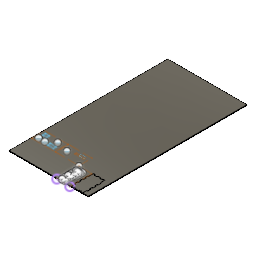
generated POWER BOX  6 CUT first v1 (Autodesk Fusion 360 design; units mm, degrees)
Autodesk Fusion 360 part; units mm, degrees
sketch "b top content" plane through (0, 0, 0) normal (0, 0, 1) x (1, 0, 0)
  line L0 (0, 85) -> (90, 85) construction
  line L1 (90, 0) -> (0, 0) construction
  line L2 (14.1663, 44.1604) -> (78.1663, 44.1604) construction
  line L3 (78.1663, 44.1604) -> (78.1663, 63.1604) construction
  line L4 (78.1663, 63.1604) -> (14.1663, 63.1604) construction
  line L5 (14.1663, 63.1604) -> (14.1663, 44.1604) construction
  line L6 (0, 0) -> (0, 85) construction
  dimension "d1818" = 15
  dimension "d1163" = 90
  dimension "d1817" = 85
  constraint horizontal L0
  constraint perpendicular L1 L6
  measures "d1163" distance of L0.start L0.end
  measures "d1817" distance of L1.start L0.end
sketch "b front content" plane through (0, 0, 0) normal (0, 0, 1) x (1, 0, 0)
  line L0 (53.5, 95.01) -> (53.5, 105.31)
  circle A0 centre (13, 101.01) radius 6
  circle A1 centre (37, 101.01) radius 6
  line L1 (76.2, 105.31) -> (76.2, 95.01)
  line L2 (26.5, 128.31) -> (26.5, 118.01)
  line L3 (26.5, 118.01) -> (12, 118.01)
  line L4 (90, 137.01) -> (0, 137.01) construction
  circle A2 centre (65, 122.51) radius 3.5
  line L5 (76.2, 95.01) -> (53.5, 95.01)
  line L6 (53.5, 105.31) -> (76.2, 105.31)
  line L7 (90, 87.01) -> (90, 137.01) construction
  line L8 (0, 87.01) -> (0, 137.01) construction
  line L9 (12, 128.31) -> (26.5, 128.31)
  line L10 (12, 118.01) -> (12, 128.31)
  line L11 (0, 87.01) -> (90, 87.01) construction
  dimension "d230" = 90
  dimension "d231" = 50
  dimension "d232" = 12
  dimension "d233" = 24
  dimension "d234" = 14
  dimension "d235" = 13
  dimension "d236" = 14.5
  dimension "d237" = 10.3
  dimension "d238" = 31
  dimension "d239" = 12
  dimension "d240" = 7
  dimension "d241" = 25
  dimension "d242" = 14.5
  dimension "d243" = 22.7
  dimension "d244" = 10.3
  dimension "d245" = 13.8
  dimension "d246" = 8
  constraint perpendicular L4 L8
  constraint equal A0 A1
  measures "d230" distance of L7.start L8.start
  measures "d231" distance of L8.start L4.end
  measures "d232" diameter of A1
  measures "d233" distance of A1.centre A0.centre
  measures "d234" distance of A1.centre L11
  measures "d235" distance of A0.centre L8
  measures "d236" distance of L2.end L3.end
  measures "d237" distance of L2.end L2.start
  measures "d238" distance of L3 L11
  measures "d239" distance of L8 L10
  measures "d240" diameter of A2
  measures "d241" distance of A2.centre L7
  measures "d242" distance of A2.centre L4
  measures "d243" distance of L1.end L0.start
  measures "d244" distance of L1.start L1.end
  measures "d245" distance of L1 L7
  measures "d246" distance of L5 L11
sketch " b back content" plane through (0, 0, 0) normal (0, 0, 1) x (1, 0, 0)
  line L0 (182.01, 87.01) -> (182.01, 137.01) construction
  line L1 (182.01, 137.01) -> (92.01, 137.01) construction
  circle A0 centre (110.81, 112.01) radius 4
  line L2 (92.01, 137.01) -> (92.01, 87.01) construction
  line L3 (169.3373, 123.3571) -> (135.0459, 123.3571) construction
  line L4 (135.0459, 123.3571) -> (135.0459, 117.5676) construction
  line L5 (135.0459, 117.5676) -> (169.3373, 117.5676) construction
  line L6 (169.3373, 117.5676) -> (169.3373, 123.3571) construction
  line L7 (92.01, 87.01) -> (182.01, 87.01) construction
  point P0 (184.02, 85)
  dimension "d1816" = 5
  dimension "d502" = 90
  dimension "d503" = 50
  dimension "d696" = 25
  dimension "d1179" = 18.8
  dimension "d1562" = 8
  measures "d502" distance of L1.end L0.end
  measures "d503" distance of L0.start L0.end
  measures "d696" distance of A0.centre L1
  measures "d1179" distance of A0.centre L2
  measures "d1562" diameter of A0
sketch "b  stock" plane through (0, 0, 0) normal (0, 0, 1) x (1, 0, 0)
  line L0 (0, 0) -> (304.8, 0)
  line L1 (304.8, 0) -> (304.8, 609.6)
  line L2 (304.8, 609.6) -> (0, 609.6)
  line L3 (0, 609.6) -> (0, 0)
extrude "b  stock body extrude Feature" add sketch "b  stock" along normal blind 3.175 makes body 1
sketch "b  layout" plane through (0, 0, 0) normal (0, 0, 1) x (1, 0, 0)
  line L0 (0, 0) -> (90, 0)
  line L1 (90, 0) -> (90, 85)
  line L2 (90, 85) -> (0, 85)
  line L3 (0, 85) -> (0, 0)
  line L4 (92.01, 0) -> (182.01, 0)
  line L5 (182.01, 0) -> (182.01, 85)
  line L6 (182.01, 85) -> (92.01, 85)
  line L7 (92.01, 85) -> (92.01, 0)
  line L8 (184.02, 0) -> (234.02, 0)
  line L9 (234.02, 0) -> (234.02, 85)
  line L10 (234.02, 85) -> (184.02, 85)
  line L11 (184.02, 85) -> (184.02, 0)
  line L12 (236.03, 0) -> (286.03, 0)
  line L13 (286.03, 0) -> (286.03, 85)
  line L14 (286.03, 85) -> (236.03, 85)
  line L15 (236.03, 85) -> (236.03, 0)
  line L16 (0, 87.01) -> (90, 87.01)
  line L17 (90, 87.01) -> (90, 137.01)
  line L18 (90, 137.01) -> (0, 137.01)
  line L19 (0, 137.01) -> (0, 87.01)
  line L20 (92.01, 87.01) -> (182.01, 87.01)
  line L21 (182.01, 87.01) -> (182.01, 137.01)
  line L22 (182.01, 137.01) -> (92.01, 137.01)
  line L23 (92.01, 137.01) -> (92.01, 87.01)
sketch "b top lines" plane through (0, 0, 0) normal (0, 0, 1) x (1, 0, 0)
  line L0 (0, 0) -> (10.15, 0)
  line L1 (10.15, 0) -> (10.15, 3.175)
  line L2 (10.15, 3.175) -> (19.85, 3.175)
  line L3 (19.85, 3.175) -> (19.85, 0)
  line L4 (19.85, 0) -> (30.15, 0)
  line L5 (30.15, 0) -> (30.15, 3.175)
  line L6 (30.15, 3.175) -> (39.85, 3.175)
  line L7 (39.85, 3.175) -> (39.85, 0)
  line L8 (39.85, 0) -> (50.15, 0)
  line L9 (50.15, 0) -> (50.15, 3.175)
  line L10 (50.15, 3.175) -> (59.85, 3.175)
  line L11 (59.85, 3.175) -> (59.85, 0)
  line L12 (59.85, 0) -> (70.15, 0)
  line L13 (70.15, 0) -> (70.15, 3.175)
  line L14 (70.15, 3.175) -> (79.85, 3.175)
  line L15 (79.85, 3.175) -> (79.85, 0)
  line L16 (79.85, 0) -> (90, 0)
  line L17 (90, 0) -> (90, 17.65)
  line L18 (90, 17.65) -> (86.825, 17.65)
  line L19 (86.825, 17.65) -> (86.825, 27.35)
  line L20 (86.825, 27.35) -> (90, 27.35)
  line L21 (90, 27.35) -> (90, 37.65)
  line L22 (90, 37.65) -> (86.825, 37.65)
  line L23 (86.825, 37.65) -> (86.825, 47.35)
  line L24 (86.825, 47.35) -> (90, 47.35)
  line L25 (90, 47.35) -> (90, 57.65)
  line L26 (90, 57.65) -> (86.825, 57.65)
  line L27 (86.825, 57.65) -> (86.825, 67.35)
  line L28 (86.825, 67.35) -> (90, 67.35)
  line L29 (90, 67.35) -> (90, 85)
  line L30 (0, 85) -> (10.15, 85)
  line L31 (10.15, 85) -> (10.15, 81.825)
  line L32 (10.15, 81.825) -> (19.85, 81.825)
  line L33 (19.85, 81.825) -> (19.85, 85)
  line L34 (19.85, 85) -> (30.15, 85)
  line L35 (30.15, 85) -> (30.15, 81.825)
  line L36 (30.15, 81.825) -> (39.85, 81.825)
  line L37 (39.85, 81.825) -> (39.85, 85)
  line L38 (39.85, 85) -> (50.15, 85)
  line L39 (50.15, 85) -> (50.15, 81.825)
  line L40 (50.15, 81.825) -> (59.85, 81.825)
  line L41 (59.85, 81.825) -> (59.85, 85)
  line L42 (59.85, 85) -> (70.15, 85)
  line L43 (70.15, 85) -> (70.15, 81.825)
  line L44 (70.15, 81.825) -> (79.85, 81.825)
  line L45 (79.85, 81.825) -> (79.85, 85)
  line L46 (79.85, 85) -> (90, 85)
  line L47 (0, 0) -> (0, 17.65)
  line L48 (0, 17.65) -> (3.175, 17.65)
  line L49 (3.175, 17.65) -> (3.175, 27.35)
  line L50 (3.175, 27.35) -> (0, 27.35)
  line L51 (0, 27.35) -> (0, 37.65)
  line L52 (0, 37.65) -> (3.175, 37.65)
  line L53 (3.175, 37.65) -> (3.175, 47.35)
  line L54 (3.175, 47.35) -> (0, 47.35)
  line L55 (0, 47.35) -> (0, 57.65)
  line L56 (0, 57.65) -> (3.175, 57.65)
  line L57 (3.175, 57.65) -> (3.175, 67.35)
  line L58 (3.175, 67.35) -> (0, 67.35)
  line L59 (0, 67.35) -> (0, 85)
sketch "b top circles" plane through (0, 0, 0) normal (0, 0, 1) x (1, 0, 0)
  circle A0 centre (10.6806, 2.4644) radius 1.005
  circle A1 centre (19.3194, 2.4644) radius 1.005
  circle A2 centre (30.6806, 2.4644) radius 1.005
  circle A3 centre (39.3194, 2.4644) radius 1.005
  circle A4 centre (50.6806, 2.4644) radius 1.005
  circle A5 centre (59.3194, 2.4644) radius 1.005
  circle A6 centre (70.6806, 2.4644) radius 1.005
  circle A7 centre (79.3194, 2.4644) radius 1.005
  circle A8 centre (87.5356, 18.1806) radius 1.005
  circle A9 centre (87.5356, 26.8194) radius 1.005
  circle A10 centre (87.5356, 38.1806) radius 1.005
  circle A11 centre (87.5356, 46.8194) radius 1.005
  circle A12 centre (87.5356, 58.1806) radius 1.005
  circle A13 centre (87.5356, 66.8194) radius 1.005
  circle A14 centre (10.6806, 82.5356) radius 1.005
  circle A15 centre (19.3194, 82.5356) radius 1.005
  circle A16 centre (30.6806, 82.5356) radius 1.005
  circle A17 centre (39.3194, 82.5356) radius 1.005
  circle A18 centre (50.6806, 82.5356) radius 1.005
  circle A19 centre (59.3194, 82.5356) radius 1.005
  circle A20 centre (70.6806, 82.5356) radius 1.005
  circle A21 centre (79.3194, 82.5356) radius 1.005
  circle A22 centre (2.4644, 18.1806) radius 1.005
  circle A23 centre (2.4644, 26.8194) radius 1.005
  circle A24 centre (2.4644, 38.1806) radius 1.005
  circle A25 centre (2.4644, 46.8194) radius 1.005
  circle A26 centre (2.4644, 58.1806) radius 1.005
  circle A27 centre (2.4644, 66.8194) radius 1.005
extrude "b top lines lines extrude Feature" add sketch "b top lines" along normal blind 3.175 separate body makes body 2
extrude "b top circles circles extrude Feature" add sketch "b top circles" along normal blind 3.175 separate body makes body 3 at (3.4644, 58.0806, 2.1167) makes body 4 at (3.4644, 38.0806, 2.1167) makes body 5 at (3.4644, 18.0806, 2.1167) makes body 6 at (69.7363, 82.8794, 2.1167) makes body 7 at (49.7363, 82.8794, 2.1167) makes body 8 at (31.6067, 82.926, 2.1167) makes body 9 at (9.7363, 82.8794, 2.1167) makes body 10 at (86.5913, 67.1631, 2.1167) makes body 11 at (87.2156, 45.8667, 1.0583) makes body 12 at (87.2156, 25.8667, 1.0583) makes body 13 at (78.9993, 1.5117, 1.0583) makes body 14 at (59.2943, 3.469, 2.1167) makes body 15 at (39.2943, 3.469, 2.1167) makes body 16 at (20.3194, 2.3643, 2.1167) makes body 17 at (31.6806, 2.3643, 2.1167) makes body 18 at (50.6556, 3.469, 2.1167) makes body 19 at (70.3606, 1.5117, 1.0583) makes body 20 at (87.2156, 17.228, 1.0583) makes body 21 at (87.2156, 37.228, 1.0583) makes body 22 at (87.2156, 57.228, 1.0583) makes body 23 at (11.6806, 2.3643, 2.1167) makes body 24 at (20.2454, 82.926, 2.1167) makes body 25 at (38.375, 82.8794, 2.1167) makes body 26 at (58.375, 82.8794, 2.1167) makes body 27 at (78.375, 82.8794, 2.1167) makes body 28 at (3.4644, 26.7193, 2.1167) makes body 29 at (3.4644, 46.7193, 2.1167) makes body 30 at (3.3904, 67.2097, 2.1167)
combine "b top lines final combine feature" operation cut target body 2 tool bodies 3 4 5 6 7 8 9 10 11 12 13 14 15 16 17 18 19 20 21 22 23 24 25 26 27 28 29 30
sketch "b bottom lines" plane through (0, 0, 0) normal (0, 0, 1) x (1, 0, 0)
  line L0 (92.01, 0) -> (102.16, 0)
  line L1 (102.16, 0) -> (102.16, 3.175)
  line L2 (102.16, 3.175) -> (111.86, 3.175)
  line L3 (111.86, 3.175) -> (111.86, 0)
  line L4 (111.86, 0) -> (122.16, 0)
  line L5 (122.16, 0) -> (122.16, 3.175)
  line L6 (122.16, 3.175) -> (131.86, 3.175)
  line L7 (131.86, 3.175) -> (131.86, 0)
  line L8 (131.86, 0) -> (142.16, 0)
  line L9 (142.16, 0) -> (142.16, 3.175)
  line L10 (142.16, 3.175) -> (151.86, 3.175)
  line L11 (151.86, 3.175) -> (151.86, 0)
  line L12 (151.86, 0) -> (162.16, 0)
  line L13 (162.16, 0) -> (162.16, 3.175)
  line L14 (162.16, 3.175) -> (171.86, 3.175)
  line L15 (171.86, 3.175) -> (171.86, 0)
  line L16 (171.86, 0) -> (182.01, 0)
  line L17 (182.01, 0) -> (182.01, 17.65)
  line L18 (182.01, 17.65) -> (178.835, 17.65)
  line L19 (178.835, 17.65) -> (178.835, 27.35)
  line L20 (178.835, 27.35) -> (182.01, 27.35)
  line L21 (182.01, 27.35) -> (182.01, 37.65)
  line L22 (182.01, 37.65) -> (178.835, 37.65)
  line L23 (178.835, 37.65) -> (178.835, 47.35)
  line L24 (178.835, 47.35) -> (182.01, 47.35)
  line L25 (182.01, 47.35) -> (182.01, 57.65)
  line L26 (182.01, 57.65) -> (178.835, 57.65)
  line L27 (178.835, 57.65) -> (178.835, 67.35)
  line L28 (178.835, 67.35) -> (182.01, 67.35)
  line L29 (182.01, 67.35) -> (182.01, 85)
  line L30 (92.01, 85) -> (102.16, 85)
  line L31 (102.16, 85) -> (102.16, 81.825)
  line L32 (102.16, 81.825) -> (111.86, 81.825)
  line L33 (111.86, 81.825) -> (111.86, 85)
  line L34 (111.86, 85) -> (122.16, 85)
  line L35 (122.16, 85) -> (122.16, 81.825)
  line L36 (122.16, 81.825) -> (131.86, 81.825)
  line L37 (131.86, 81.825) -> (131.86, 85)
  line L38 (131.86, 85) -> (142.16, 85)
  line L39 (142.16, 85) -> (142.16, 81.825)
  line L40 (142.16, 81.825) -> (151.86, 81.825)
  line L41 (151.86, 81.825) -> (151.86, 85)
  line L42 (151.86, 85) -> (162.16, 85)
  line L43 (162.16, 85) -> (162.16, 81.825)
  line L44 (162.16, 81.825) -> (171.86, 81.825)
  line L45 (171.86, 81.825) -> (171.86, 85)
  line L46 (171.86, 85) -> (182.01, 85)
  line L47 (92.01, 0) -> (92.01, 17.65)
  line L48 (92.01, 17.65) -> (95.185, 17.65)
  line L49 (95.185, 17.65) -> (95.185, 27.35)
  line L50 (95.185, 27.35) -> (92.01, 27.35)
  line L51 (92.01, 27.35) -> (92.01, 37.65)
  line L52 (92.01, 37.65) -> (95.185, 37.65)
  line L53 (95.185, 37.65) -> (95.185, 47.35)
  line L54 (95.185, 47.35) -> (92.01, 47.35)
  line L55 (92.01, 47.35) -> (92.01, 57.65)
  line L56 (92.01, 57.65) -> (95.185, 57.65)
  line L57 (95.185, 57.65) -> (95.185, 67.35)
  line L58 (95.185, 67.35) -> (92.01, 67.35)
  line L59 (92.01, 67.35) -> (92.01, 85)
sketch "b bottom circles" plane through (0, 0, 0) normal (0, 0, 1) x (1, 0, 0)
  circle A0 centre (102.6906, 2.4644) radius 1.005
  circle A1 centre (111.3294, 2.4644) radius 1.005
  circle A2 centre (122.6906, 2.4644) radius 1.005
  circle A3 centre (131.3294, 2.4644) radius 1.005
  circle A4 centre (142.6906, 2.4644) radius 1.005
  circle A5 centre (151.3294, 2.4644) radius 1.005
  circle A6 centre (162.6906, 2.4644) radius 1.005
  circle A7 centre (171.3294, 2.4644) radius 1.005
  circle A8 centre (179.5456, 18.1806) radius 1.005
  circle A9 centre (179.5456, 26.8194) radius 1.005
  circle A10 centre (179.5456, 38.1806) radius 1.005
  circle A11 centre (179.5456, 46.8194) radius 1.005
  circle A12 centre (179.5456, 58.1806) radius 1.005
  circle A13 centre (179.5456, 66.8194) radius 1.005
  circle A14 centre (102.6906, 82.5356) radius 1.005
  circle A15 centre (111.3294, 82.5356) radius 1.005
  circle A16 centre (122.6906, 82.5356) radius 1.005
  circle A17 centre (131.3294, 82.5356) radius 1.005
  circle A18 centre (142.6906, 82.5356) radius 1.005
  circle A19 centre (151.3294, 82.5356) radius 1.005
  circle A20 centre (162.6906, 82.5356) radius 1.005
  circle A21 centre (171.3294, 82.5356) radius 1.005
  circle A22 centre (94.4744, 18.1806) radius 1.005
  circle A23 centre (94.4744, 26.8194) radius 1.005
  circle A24 centre (94.4744, 38.1806) radius 1.005
  circle A25 centre (94.4744, 46.8194) radius 1.005
  circle A26 centre (94.4744, 58.1806) radius 1.005
  circle A27 centre (94.4744, 66.8194) radius 1.005
sketch "b bottom content" plane through (0, 0, 0) normal (0, 0, 1) x (1, 0, 0)
  line L0 (92.01, 0) -> (182.01, 0) construction
  line L1 (182.01, 0) -> (182.01, 85) construction
  line L2 (182.01, 85) -> (92.01, 85) construction
  line L3 (92.01, 85) -> (92.01, 0) construction
  line L4 (182.01, 85) -> (182.01, 0) construction
  line L5 (182.01, 0) -> (92.01, 0) construction
  line L6 (92.01, 85) -> (182.01, 85) construction
  line L7 (92.01, 0) -> (92.01, 85) construction
  circle A0 centre (108.01, 55.5) radius 1.005
  circle A1 centre (172.01, 75) radius 1.005
  circle A2 centre (166.01, 55.5) radius 1.005
  circle A3 centre (166.01, 29.5) radius 1.005
  circle A4 centre (172.01, 10) radius 1.005
  circle A5 centre (102.01, 10) radius 1.005
  circle A6 centre (108.01, 29.5) radius 1.005
  circle A7 centre (102.01, 75) radius 1.005
  circle A8 centre (172.01, 75) radius 1.005
  point P0 (102.01, 75)
  point P1 (108.01, 55.5)
  point P2 (172.01, 75)
  point P3 (166.01, 29.5)
  point P4 (166.01, 55.5)
  point P5 (172.01, 10)
  point P6 (102.01, 10)
  point P7 (108.01, 29.5)
  point P8 (182.01, 85)
  dimension "d467" = 90
  dimension "d468" = 85
  dimension "d469" = 10
  dimension "d470" = 10
  dimension "d471" = 29.5
  dimension "d472" = 16
  dimension "d473" = 2.01
  dimension "d474" = 2.01
  constraint horizontal L5
  constraint perpendicular L5 L7
  constraint parallel L5 L6
  constraint coincident L1.end L2.start
  constraint vertical L4
  constraint coincident P1 A0.centre
  constraint coincident P2 A1.centre
  constraint coincident P4 A2.centre
  constraint coincident P3 A3.centre
  constraint coincident P5 A4.centre
  constraint coincident P6 A5.centre
  constraint coincident P7 A6.centre
  constraint coincident P0 A7.centre
  constraint concentric A1 A8
  constraint equal A0 A2
  constraint equal A7 A8
  constraint equal A0 A6
  constraint equal A0 A3
  constraint equal A3 A5
  constraint equal A3 A8
  constraint equal A2 A4
  measures "d467" distance of L1.end L2.end
  measures "d468" distance of L0.start L2.end
  measures "d469" distance of P0 L6
  measures "d470" distance of P0 L7
  measures "d471" distance of P1 L6
  measures "d472" distance of P7 L7
  measures "d473" diameter of A0
  measures "d474" diameter of A1
extrude "b bottom lines lines extrude Feature" add sketch "b bottom lines" along normal blind 3.175 separate body makes body 31
extrude "b bottom circles circles extrude Feature" add sketch "b bottom circles" along normal blind 3.175 separate body makes body 32 at (94.1543, 57.228, 1.0583) makes body 33 at (94.1543, 37.228, 1.0583) makes body 34 at (94.1543, 17.228, 1.0583) makes body 35 at (161.7463, 82.8794, 2.1167) makes body 36 at (141.7463, 82.8794, 2.1167) makes body 37 at (121.7463, 82.8794, 2.1167) makes body 38 at (101.7463, 82.8794, 2.1167) makes body 39 at (178.6013, 67.1631, 2.1167) makes body 40 at (180.4717, 47.2097, 2.1167) makes body 41 at (179.959, 27.7354, 2.1167) makes body 42 at (170.916, 3.3804, 2.1167) makes body 43 at (150.916, 3.3804, 2.1167) makes body 44 at (130.916, 3.3804, 2.1167) makes body 45 at (111.0093, 1.5117, 1.0583) makes body 46 at (122.3706, 1.5117, 1.0583) makes body 47 at (142.2773, 3.3804, 2.1167) makes body 48 at (162.2773, 3.3804, 2.1167) makes body 49 at (179.959, 19.0967, 2.1167) makes body 50 at (180.4717, 38.571, 2.1167) makes body 51 at (180.4717, 58.571, 2.1167) makes body 52 at (102.3706, 1.5117, 1.0583) makes body 53 at (110.385, 82.8794, 2.1167) makes body 54 at (130.385, 82.8794, 2.1167) makes body 55 at (150.385, 82.8794, 2.1167) makes body 56 at (170.385, 82.8794, 2.1167) makes body 57 at (94.1543, 25.8667, 1.0583) makes body 58 at (94.1543, 45.8667, 1.0583) makes body 59 at (93.53, 67.1631, 2.1167)
combine "b bottom lines final combine feature" operation cut target body 31 tool bodies 32 33 34 35 36 37 38 39 40 41 42 43 44 45 46 47 48 49 50 51 52 53 54 55 56 57 58 59
sketch "b left lines" plane through (0, 0, 0) normal (0, 0, 1) x (1, 0, 0)
  line L0 (187.195, 0) -> (194.17, 0)
  line L1 (194.17, 0) -> (194.17, 3.175)
  line L2 (194.17, 3.175) -> (203.87, 3.175)
  line L3 (203.87, 3.175) -> (203.87, 0)
  line L4 (203.87, 0) -> (214.17, 0)
  line L5 (214.17, 0) -> (214.17, 3.175)
  line L6 (214.17, 3.175) -> (223.87, 3.175)
  line L7 (223.87, 3.175) -> (223.87, 0)
  line L8 (223.87, 0) -> (230.845, 0)
  line L9 (230.845, 0) -> (230.845, 17.35)
  line L10 (230.845, 17.35) -> (234.02, 17.35)
  line L11 (234.02, 17.35) -> (234.02, 27.65)
  line L12 (234.02, 27.65) -> (230.845, 27.65)
  line L13 (230.845, 27.65) -> (230.845, 37.35)
  line L14 (230.845, 37.35) -> (234.02, 37.35)
  line L15 (234.02, 37.35) -> (234.02, 47.65)
  line L16 (234.02, 47.65) -> (230.845, 47.65)
  line L17 (230.845, 47.65) -> (230.845, 57.35)
  line L18 (230.845, 57.35) -> (234.02, 57.35)
  line L19 (234.02, 57.35) -> (234.02, 67.65)
  line L20 (234.02, 67.65) -> (230.845, 67.65)
  line L21 (230.845, 67.65) -> (230.845, 85)
  line L22 (187.195, 85) -> (194.17, 85)
  line L23 (194.17, 85) -> (194.17, 81.825)
  line L24 (194.17, 81.825) -> (203.87, 81.825)
  line L25 (203.87, 81.825) -> (203.87, 85)
  line L26 (203.87, 85) -> (214.17, 85)
  line L27 (214.17, 85) -> (214.17, 81.825)
  line L28 (214.17, 81.825) -> (223.87, 81.825)
  line L29 (223.87, 81.825) -> (223.87, 85)
  line L30 (223.87, 85) -> (230.845, 85)
  line L31 (187.195, 0) -> (187.195, 17.35)
  line L32 (187.195, 17.35) -> (184.02, 17.35)
  line L33 (184.02, 17.35) -> (184.02, 27.65)
  line L34 (184.02, 27.65) -> (187.195, 27.65)
  line L35 (187.195, 27.65) -> (187.195, 37.35)
  line L36 (187.195, 37.35) -> (184.02, 37.35)
  line L37 (184.02, 37.35) -> (184.02, 47.65)
  line L38 (184.02, 47.65) -> (187.195, 47.65)
  line L39 (187.195, 47.65) -> (187.195, 57.35)
  line L40 (187.195, 57.35) -> (184.02, 57.35)
  line L41 (184.02, 57.35) -> (184.02, 67.65)
  line L42 (184.02, 67.65) -> (187.195, 67.65)
  line L43 (187.195, 67.65) -> (187.195, 85)
sketch "b left circles" plane through (0, 0, 0) normal (0, 0, 1) x (1, 0, 0)
  circle A0 centre (194.7006, 2.4644) radius 1.005
  circle A1 centre (203.3394, 2.4644) radius 1.005
  circle A2 centre (214.7006, 2.4644) radius 1.005
  circle A3 centre (223.3394, 2.4644) radius 1.005
  circle A4 centre (231.5556, 16.8194) radius 1.005
  circle A5 centre (231.5556, 28.1806) radius 1.005
  circle A6 centre (231.5556, 36.8194) radius 1.005
  circle A7 centre (231.5556, 48.1806) radius 1.005
  circle A8 centre (231.5556, 56.8194) radius 1.005
  circle A9 centre (231.5556, 68.1806) radius 1.005
  circle A10 centre (194.7006, 82.5356) radius 1.005
  circle A11 centre (203.3394, 82.5356) radius 1.005
  circle A12 centre (214.7006, 82.5356) radius 1.005
  circle A13 centre (223.3394, 82.5356) radius 1.005
  circle A14 centre (186.4844, 16.8194) radius 1.005
  circle A15 centre (186.4844, 28.1806) radius 1.005
  circle A16 centre (186.4844, 36.8194) radius 1.005
  circle A17 centre (186.4844, 48.1806) radius 1.005
  circle A18 centre (186.4844, 56.8194) radius 1.005
  circle A19 centre (186.4844, 68.1806) radius 1.005
sketch "b left content" plane through (0, 0, 0) normal (0, 0, 1) x (1, 0, 0)
  line L0 (184.02, 0) -> (234.02, 0) construction
  line L1 (234.02, 0) -> (234.02, 85) construction
  line L2 (234.02, 85) -> (184.02, 85) construction
  line L3 (184.02, 85) -> (184.02, 0) construction
  circle A0 centre (205.99, 40) radius 1.5
  circle A1 centre (205.99, 52) radius 1.5
  circle A2 centre (193.99, 52) radius 1.5
  circle A3 centre (193.99, 64) radius 1.5
  circle A4 centre (205.99, 64) radius 0
  circle A5 centre (199.99, 16) radius 1.5
  circle A6 centre (199.99, 52) radius 1.5
  circle A7 centre (199.99, 64) radius 0
  circle A8 centre (199.99, 46) radius 1.5
  circle A9 centre (193.99, 28) radius 1.5
  circle A10 centre (199.99, 22) radius 1.5
  circle A11 centre (205.99, 28) radius 1.5
  circle A12 centre (199.99, 28) radius 1.5
  circle A13 centre (193.99, 58) radius 1.5
  circle A14 centre (205.99, 22) radius 1.5
  circle A15 centre (205.99, 10) radius 1.5
  circle A16 centre (193.99, 22) radius 1.5
  circle A17 centre (205.99, 34) radius 1.5
  circle A18 centre (193.99, 34) radius 1.5
  circle A19 centre (199.99, 58) radius 1.5
  circle A20 centre (193.99, 16) radius 1.5
  circle A21 centre (199.99, 10) radius 1.5
  circle A22 centre (193.99, 64) radius 0
  circle A23 centre (199.99, 34) radius 1.5
  circle A24 centre (199.99, 64) radius 1.5
  circle A25 centre (205.99, 46) radius 1.5
  circle A26 centre (193.99, 10) radius 1.5
  circle A27 centre (193.99, 46) radius 1.5
  circle A28 centre (193.99, 40) radius 1.5
  circle A29 centre (205.99, 58) radius 1.5
  circle A30 centre (205.99, 16) radius 1.5
  circle A31 centre (199.99, 40) radius 1.5
  circle A32 centre (205.99, 64) radius 1.5
  line L4 (184.02, 0) -> (234.02, 0)
  point P0 (193.99, 70)
  point P1 (199.99, 70)
  point P2 (211.99, 46)
  point P3 (211.99, 52)
  point P4 (211.99, 64)
  point P5 (205.99, 70)
  point P6 (211.99, 58)
  point P7 (211.99, 70)
  point P8 (194.02, 10)
  dimension "d487" = 6
  dimension "d488" = 6
  dimension "d489" = 10
  dimension "d490" = 10
  measures "d489" distance of L3 P8
  measures "d490" distance of A26.centre L4
extrude "b left lines lines extrude Feature" add sketch "b left lines" along normal blind 3.175 separate body makes body 60
extrude "b left circles circles extrude Feature" add sketch "b left circles" along normal blind 3.175 separate body makes body 61 at (187.4104, 57.2097, 2.1167) makes body 62 at (187.4104, 37.2097, 2.1167) makes body 63 at (186.8977, 17.7354, 2.1167) makes body 64 at (213.7563, 82.8794, 2.1167) makes body 65 at (193.7563, 82.8794, 2.1167) makes body 66 at (230.6113, 68.5244, 2.1167) makes body 67 at (232.4817, 48.571, 2.1167) makes body 68 at (231.969, 29.0967, 2.1167) makes body 69 at (222.926, 3.3804, 2.1167) makes body 70 at (202.926, 3.3804, 2.1167) makes body 71 at (214.2873, 3.3804, 2.1167) makes body 72 at (231.969, 17.7354, 2.1167) makes body 73 at (232.4817, 37.2097, 2.1167) makes body 74 at (232.4817, 57.2097, 2.1167) makes body 75 at (194.2873, 3.3804, 2.1167) makes body 76 at (202.395, 82.8794, 2.1167) makes body 77 at (222.395, 82.8794, 2.1167) makes body 78 at (186.8977, 29.0967, 2.1167) makes body 79 at (187.4104, 48.571, 2.1167) makes body 80 at (185.54, 68.5244, 2.1167)
combine "b left lines final combine feature" operation cut target body 60 tool bodies 61 62 63 64 65 66 67 68 69 70 71 72 73 74 75 76 77 78 79 80
sketch "b right lines" plane through (0, 0, 0) normal (0, 0, 1) x (1, 0, 0)
  line L0 (239.205, 0) -> (246.18, 0)
  line L1 (246.18, 0) -> (246.18, 3.175)
  line L2 (246.18, 3.175) -> (255.88, 3.175)
  line L3 (255.88, 3.175) -> (255.88, 0)
  line L4 (255.88, 0) -> (266.18, 0)
  line L5 (266.18, 0) -> (266.18, 3.175)
  line L6 (266.18, 3.175) -> (275.88, 3.175)
  line L7 (275.88, 3.175) -> (275.88, 0)
  line L8 (275.88, 0) -> (282.855, 0)
  line L9 (282.855, 0) -> (282.855, 17.35)
  line L10 (282.855, 17.35) -> (286.03, 17.35)
  line L11 (286.03, 17.35) -> (286.03, 27.65)
  line L12 (286.03, 27.65) -> (282.855, 27.65)
  line L13 (282.855, 27.65) -> (282.855, 37.35)
  line L14 (282.855, 37.35) -> (286.03, 37.35)
  line L15 (286.03, 37.35) -> (286.03, 47.65)
  line L16 (286.03, 47.65) -> (282.855, 47.65)
  line L17 (282.855, 47.65) -> (282.855, 57.35)
  line L18 (282.855, 57.35) -> (286.03, 57.35)
  line L19 (286.03, 57.35) -> (286.03, 67.65)
  line L20 (286.03, 67.65) -> (282.855, 67.65)
  line L21 (282.855, 67.65) -> (282.855, 85)
  line L22 (239.205, 85) -> (246.18, 85)
  line L23 (246.18, 85) -> (246.18, 81.825)
  line L24 (246.18, 81.825) -> (255.88, 81.825)
  line L25 (255.88, 81.825) -> (255.88, 85)
  line L26 (255.88, 85) -> (266.18, 85)
  line L27 (266.18, 85) -> (266.18, 81.825)
  line L28 (266.18, 81.825) -> (275.88, 81.825)
  line L29 (275.88, 81.825) -> (275.88, 85)
  line L30 (275.88, 85) -> (282.855, 85)
  line L31 (239.205, 0) -> (239.205, 17.35)
  line L32 (239.205, 17.35) -> (236.03, 17.35)
  line L33 (236.03, 17.35) -> (236.03, 27.65)
  line L34 (236.03, 27.65) -> (239.205, 27.65)
  line L35 (239.205, 27.65) -> (239.205, 37.35)
  line L36 (239.205, 37.35) -> (236.03, 37.35)
  line L37 (236.03, 37.35) -> (236.03, 47.65)
  line L38 (236.03, 47.65) -> (239.205, 47.65)
  line L39 (239.205, 47.65) -> (239.205, 57.35)
  line L40 (239.205, 57.35) -> (236.03, 57.35)
  line L41 (236.03, 57.35) -> (236.03, 67.65)
  line L42 (236.03, 67.65) -> (239.205, 67.65)
  line L43 (239.205, 67.65) -> (239.205, 85)
sketch "b right circles" plane through (0, 0, 0) normal (0, 0, 1) x (1, 0, 0)
  circle A0 centre (246.7106, 2.4644) radius 1.005
  circle A1 centre (255.3494, 2.4644) radius 1.005
  circle A2 centre (266.7106, 2.4644) radius 1.005
  circle A3 centre (275.3494, 2.4644) radius 1.005
  circle A4 centre (283.5656, 16.8194) radius 1.005
  circle A5 centre (283.5656, 28.1806) radius 1.005
  circle A6 centre (283.5656, 36.8194) radius 1.005
  circle A7 centre (283.5656, 48.1806) radius 1.005
  circle A8 centre (283.5656, 56.8194) radius 1.005
  circle A9 centre (283.5656, 68.1806) radius 1.005
  circle A10 centre (246.7106, 82.5356) radius 1.005
  circle A11 centre (255.3494, 82.5356) radius 1.005
  circle A12 centre (266.7106, 82.5356) radius 1.005
  circle A13 centre (275.3494, 82.5356) radius 1.005
  circle A14 centre (238.4944, 16.8194) radius 1.005
  circle A15 centre (238.4944, 28.1806) radius 1.005
  circle A16 centre (238.4944, 36.8194) radius 1.005
  circle A17 centre (238.4944, 48.1806) radius 1.005
  circle A18 centre (238.4944, 56.8194) radius 1.005
  circle A19 centre (238.4944, 68.1806) radius 1.005
sketch "b right content" plane through (0, 0, 0) normal (0, 0, 1) x (1, 0, 0)
  line L0 (236.03, 0) -> (286.03, 0) construction
  line L1 (286.03, 0) -> (286.03, 85) construction
  line L2 (286.03, 85) -> (236.03, 85) construction
  line L3 (236.03, 85) -> (236.03, 0) construction
  circle A0 centre (257.99, 64) radius 0
  circle A1 centre (251.99, 64) radius 0
  circle A2 centre (245.99, 64) radius 0
  circle A3 centre (246.03, 10) radius 0
  circle A4 centre (245.99, 10) radius 1.5
  circle A5 centre (263.99, 46) radius 0
  circle A6 centre (263.99, 52) radius 0
  circle A7 centre (263.99, 58) radius 0
  circle A8 centre (263.99, 64) radius 0
  circle A9 centre (245.99, 70) radius 0
  circle A10 centre (251.99, 70) radius 0
  circle A11 centre (257.99, 70) radius 0
  circle A12 centre (263.99, 70) radius 0
  circle A13 centre (251.99, 10) radius 1.5
  circle A14 centre (257.99, 10) radius 1.5
  circle A15 centre (245.99, 16) radius 1.5
  circle A16 centre (251.99, 16) radius 1.5
  circle A17 centre (257.99, 16) radius 1.5
  circle A18 centre (245.99, 22) radius 1.5
  circle A19 centre (251.99, 22) radius 1.5
  circle A20 centre (257.99, 22) radius 1.5
  circle A21 centre (245.99, 28) radius 1.5
  circle A22 centre (251.99, 28) radius 1.5
  circle A23 centre (257.99, 28) radius 1.5
  circle A24 centre (245.99, 34) radius 1.5
  circle A25 centre (251.99, 34) radius 1.5
  circle A26 centre (257.99, 34) radius 1.5
  circle A27 centre (245.99, 40) radius 1.5
  circle A28 centre (251.99, 40) radius 1.5
  circle A29 centre (257.99, 40) radius 1.5
  circle A30 centre (245.99, 46) radius 1.5
  circle A31 centre (251.99, 46) radius 1.5
  circle A32 centre (257.99, 46) radius 1.5
  circle A33 centre (245.99, 52) radius 1.5
  circle A34 centre (251.99, 52) radius 1.5
  circle A35 centre (257.99, 52) radius 1.5
  circle A36 centre (245.99, 58) radius 1.5
  circle A37 centre (251.99, 58) radius 1.5
  circle A38 centre (257.99, 58) radius 1.5
  circle A39 centre (245.99, 64) radius 1.5
  circle A40 centre (251.99, 64) radius 1.5
  circle A41 centre (257.99, 64) radius 1.5
  line L4 (236.03, 85) -> (236.03, 0)
  point P0 (-142.01, 0)
  point P1 (-117.01, 0)
  dimension "d479" = 0
  dimension "d483" = 6
  dimension "d484" = 6
  dimension "d491" = 10
  dimension "d494" = 10
  measures "d479" diameter of A3
  measures "d491" vertical distance of L0.start A3.centre
  measures "d494" distance of A3.centre L4
extrude "b right lines lines extrude Feature" add sketch "b right lines" along normal blind 3.175 separate body makes body 81
extrude "b right circles circles extrude Feature" add sketch "b right circles" along normal blind 3.175 separate body makes body 82 at (239.4204, 57.2097, 2.1167) makes body 83 at (239.4204, 37.2097, 2.1167) makes body 84 at (238.9077, 17.7354, 2.1167) makes body 85 at (266.9828, 83.5031, 2.1167) makes body 86 at (245.7663, 82.8794, 2.1167) makes body 87 at (283.8378, 69.1481, 2.1167) makes body 88 at (283.8378, 49.1481, 2.1167) makes body 89 at (283.8378, 29.1481, 2.1167) makes body 90 at (275.6216, 3.4318, 2.1167) makes body 91 at (256.1192, 3.1104, 2.1167) makes body 92 at (266.9828, 3.4318, 2.1167) makes body 93 at (283.8378, 17.7868, 2.1167) makes body 94 at (283.8378, 37.7868, 2.1167) makes body 95 at (283.8378, 57.7868, 2.1167) makes body 96 at (246.2973, 3.3804, 2.1167) makes body 97 at (254.405, 82.8794, 2.1167) makes body 98 at (275.6216, 83.5031, 2.1167) makes body 99 at (238.9077, 29.0967, 2.1167) makes body 100 at (239.4204, 48.571, 2.1167) makes body 101 at (237.55, 68.5244, 2.1167)
combine "b right lines final combine feature" operation cut target body 81 tool bodies 82 83 84 85 86 87 88 89 90 91 92 93 94 95 96 97 98 99 100 101
sketch "b front lines" plane through (0, 0, 0) normal (0, 0, 1) x (1, 0, 0)
  line L0 (3.175, 90.185) -> (9.85, 90.185)
  line L1 (9.85, 90.185) -> (9.85, 87.01)
  line L2 (9.85, 87.01) -> (20.15, 87.01)
  line L3 (20.15, 87.01) -> (20.15, 90.185)
  line L4 (20.15, 90.185) -> (29.85, 90.185)
  line L5 (29.85, 90.185) -> (29.85, 87.01)
  line L6 (29.85, 87.01) -> (40.15, 87.01)
  line L7 (40.15, 87.01) -> (40.15, 90.185)
  line L8 (40.15, 90.185) -> (49.85, 90.185)
  line L9 (49.85, 90.185) -> (49.85, 87.01)
  line L10 (49.85, 87.01) -> (60.15, 87.01)
  line L11 (60.15, 87.01) -> (60.15, 90.185)
  line L12 (60.15, 90.185) -> (69.85, 90.185)
  line L13 (69.85, 90.185) -> (69.85, 87.01)
  line L14 (69.85, 87.01) -> (80.15, 87.01)
  line L15 (80.15, 87.01) -> (80.15, 90.185)
  line L16 (80.15, 90.185) -> (86.825, 90.185)
  line L17 (86.825, 90.185) -> (86.825, 96.86)
  line L18 (86.825, 96.86) -> (90, 96.86)
  line L19 (90, 96.86) -> (90, 107.16)
  line L20 (90, 107.16) -> (86.825, 107.16)
  line L21 (86.825, 107.16) -> (86.825, 116.86)
  line L22 (86.825, 116.86) -> (90, 116.86)
  line L23 (90, 116.86) -> (90, 127.16)
  line L24 (90, 127.16) -> (86.825, 127.16)
  line L25 (86.825, 127.16) -> (86.825, 133.835)
  line L26 (3.175, 133.835) -> (9.85, 133.835)
  line L27 (9.85, 133.835) -> (9.85, 137.01)
  line L28 (9.85, 137.01) -> (20.15, 137.01)
  line L29 (20.15, 137.01) -> (20.15, 133.835)
  line L30 (20.15, 133.835) -> (29.85, 133.835)
  line L31 (29.85, 133.835) -> (29.85, 137.01)
  line L32 (29.85, 137.01) -> (40.15, 137.01)
  line L33 (40.15, 137.01) -> (40.15, 133.835)
  line L34 (40.15, 133.835) -> (49.85, 133.835)
  line L35 (49.85, 133.835) -> (49.85, 137.01)
  line L36 (49.85, 137.01) -> (60.15, 137.01)
  line L37 (60.15, 137.01) -> (60.15, 133.835)
  line L38 (60.15, 133.835) -> (69.85, 133.835)
  line L39 (69.85, 133.835) -> (69.85, 137.01)
  line L40 (69.85, 137.01) -> (80.15, 137.01)
  line L41 (80.15, 137.01) -> (80.15, 133.835)
  line L42 (80.15, 133.835) -> (86.825, 133.835)
  line L43 (3.175, 90.185) -> (3.175, 96.86)
  line L44 (3.175, 96.86) -> (0, 96.86)
  line L45 (0, 96.86) -> (0, 107.16)
  line L46 (0, 107.16) -> (3.175, 107.16)
  line L47 (3.175, 107.16) -> (3.175, 116.86)
  line L48 (3.175, 116.86) -> (0, 116.86)
  line L49 (0, 116.86) -> (0, 127.16)
  line L50 (0, 127.16) -> (3.175, 127.16)
  line L51 (3.175, 127.16) -> (3.175, 133.835)
sketch "b front circles" plane through (0, 0, 0) normal (0, 0, 1) x (1, 0, 0)
  circle A0 centre (9.3194, 89.4744) radius 1.005
  circle A1 centre (20.6806, 89.4744) radius 1.005
  circle A2 centre (29.3194, 89.4744) radius 1.005
  circle A3 centre (40.6806, 89.4744) radius 1.005
  circle A4 centre (49.3194, 89.4744) radius 1.005
  circle A5 centre (60.6806, 89.4744) radius 1.005
  circle A6 centre (69.3194, 89.4744) radius 1.005
  circle A7 centre (80.6806, 89.4744) radius 1.005
  circle A8 centre (87.5356, 96.3294) radius 1.005
  circle A9 centre (87.5356, 107.6906) radius 1.005
  circle A10 centre (87.5356, 116.3294) radius 1.005
  circle A11 centre (87.5356, 127.6906) radius 1.005
  circle A12 centre (9.3194, 134.5456) radius 1.005
  circle A13 centre (20.6806, 134.5456) radius 1.005
  circle A14 centre (29.3194, 134.5456) radius 1.005
  circle A15 centre (40.6806, 134.5456) radius 1.005
  circle A16 centre (49.3194, 134.5456) radius 1.005
  circle A17 centre (60.6806, 134.5456) radius 1.005
  circle A18 centre (69.3194, 134.5456) radius 1.005
  circle A19 centre (80.6806, 134.5456) radius 1.005
  circle A20 centre (2.4644, 96.3294) radius 1.005
  circle A21 centre (2.4644, 107.6906) radius 1.005
  circle A22 centre (2.4644, 116.3294) radius 1.005
  circle A23 centre (2.4644, 127.6906) radius 1.005
extrude "b front lines lines extrude Feature" add sketch "b front lines" along normal blind 3.175 separate body makes body 102
extrude "b front circles circles extrude Feature" add sketch "b front circles" along normal blind 3.175 separate body makes body 103 at (3.3904, 116.7197, 2.1167) makes body 104 at (3.3904, 96.7197, 2.1167) makes body 105 at (70.0892, 135.1916, 2.1167) makes body 106 at (50.0892, 135.1916, 2.1167) makes body 107 at (29.7327, 135.4617, 2.1167) makes body 108 at (8.5495, 133.8996, 2.1167) makes body 109 at (86.5913, 128.0344, 2.1167) makes body 110 at (86.5913, 108.0344, 2.1167) makes body 111 at (79.7363, 89.8181, 2.1167) makes body 112 at (59.7363, 89.8181, 2.1167) makes body 113 at (39.7363, 89.8181, 2.1167) makes body 114 at (21.6067, 89.8647, 2.1167) makes body 115 at (30.2454, 89.8647, 2.1167) makes body 116 at (48.375, 89.8181, 2.1167) makes body 117 at (68.375, 89.8181, 2.1167) makes body 118 at (86.5913, 96.6731, 2.1167) makes body 119 at (86.5913, 116.6731, 2.1167) makes body 120 at (10.2454, 89.8647, 2.1167) makes body 121 at (21.094, 135.4617, 2.1167) makes body 122 at (41.4505, 135.1916, 2.1167) makes body 123 at (61.4505, 135.1916, 2.1167) makes body 124 at (81.4505, 135.1916, 2.1167) makes body 125 at (3.3904, 108.081, 2.1167) makes body 126 at (3.3904, 128.081, 2.1167)
combine "b front lines final combine feature" operation cut target body 102 tool bodies 103 104 105 106 107 108 109 110 111 112 113 114 115 116 117 118 119 120 121 122 123 124 125 126
sketch "b back lines" plane through (0, 0, 0) normal (0, 0, 1) x (1, 0, 0)
  line L0 (95.185, 90.185) -> (101.86, 90.185)
  line L1 (101.86, 90.185) -> (101.86, 87.01)
  line L2 (101.86, 87.01) -> (112.16, 87.01)
  line L3 (112.16, 87.01) -> (112.16, 90.185)
  line L4 (112.16, 90.185) -> (121.86, 90.185)
  line L5 (121.86, 90.185) -> (121.86, 87.01)
  line L6 (121.86, 87.01) -> (132.16, 87.01)
  line L7 (132.16, 87.01) -> (132.16, 90.185)
  line L8 (132.16, 90.185) -> (141.86, 90.185)
  line L9 (141.86, 90.185) -> (141.86, 87.01)
  line L10 (141.86, 87.01) -> (152.16, 87.01)
  line L11 (152.16, 87.01) -> (152.16, 90.185)
  line L12 (152.16, 90.185) -> (161.86, 90.185)
  line L13 (161.86, 90.185) -> (161.86, 87.01)
  line L14 (161.86, 87.01) -> (172.16, 87.01)
  line L15 (172.16, 87.01) -> (172.16, 90.185)
  line L16 (172.16, 90.185) -> (178.835, 90.185)
  line L17 (178.835, 90.185) -> (178.835, 96.86)
  line L18 (178.835, 96.86) -> (182.01, 96.86)
  line L19 (182.01, 96.86) -> (182.01, 107.16)
  line L20 (182.01, 107.16) -> (178.835, 107.16)
  line L21 (178.835, 107.16) -> (178.835, 116.86)
  line L22 (178.835, 116.86) -> (182.01, 116.86)
  line L23 (182.01, 116.86) -> (182.01, 127.16)
  line L24 (182.01, 127.16) -> (178.835, 127.16)
  line L25 (178.835, 127.16) -> (178.835, 133.835)
  line L26 (95.185, 133.835) -> (101.86, 133.835)
  line L27 (101.86, 133.835) -> (101.86, 137.01)
  line L28 (101.86, 137.01) -> (112.16, 137.01)
  line L29 (112.16, 137.01) -> (112.16, 133.835)
  line L30 (112.16, 133.835) -> (121.86, 133.835)
  line L31 (121.86, 133.835) -> (121.86, 137.01)
  line L32 (121.86, 137.01) -> (132.16, 137.01)
  line L33 (132.16, 137.01) -> (132.16, 133.835)
  line L34 (132.16, 133.835) -> (141.86, 133.835)
  line L35 (141.86, 133.835) -> (141.86, 137.01)
  line L36 (141.86, 137.01) -> (152.16, 137.01)
  line L37 (152.16, 137.01) -> (152.16, 133.835)
  line L38 (152.16, 133.835) -> (161.86, 133.835)
  line L39 (161.86, 133.835) -> (161.86, 137.01)
  line L40 (161.86, 137.01) -> (172.16, 137.01)
  line L41 (172.16, 137.01) -> (172.16, 133.835)
  line L42 (172.16, 133.835) -> (178.835, 133.835)
  line L43 (95.185, 90.185) -> (95.185, 96.86)
  line L44 (95.185, 96.86) -> (92.01, 96.86)
  line L45 (92.01, 96.86) -> (92.01, 107.16)
  line L46 (92.01, 107.16) -> (95.185, 107.16)
  line L47 (95.185, 107.16) -> (95.185, 116.86)
  line L48 (95.185, 116.86) -> (92.01, 116.86)
  line L49 (92.01, 116.86) -> (92.01, 127.16)
  line L50 (92.01, 127.16) -> (95.185, 127.16)
  line L51 (95.185, 127.16) -> (95.185, 133.835)
sketch "b back circles" plane through (0, 0, 0) normal (0, 0, 1) x (1, 0, 0)
  circle A0 centre (101.3294, 89.4744) radius 1.005
  circle A1 centre (112.6906, 89.4744) radius 1.005
  circle A2 centre (121.3294, 89.4744) radius 1.005
  circle A3 centre (132.6906, 89.4744) radius 1.005
  circle A4 centre (141.3294, 89.4744) radius 1.005
  circle A5 centre (152.6906, 89.4744) radius 1.005
  circle A6 centre (161.3294, 89.4744) radius 1.005
  circle A7 centre (172.6906, 89.4744) radius 1.005
  circle A8 centre (179.5456, 96.3294) radius 1.005
  circle A9 centre (179.5456, 107.6906) radius 1.005
  circle A10 centre (179.5456, 116.3294) radius 1.005
  circle A11 centre (179.5456, 127.6906) radius 1.005
  circle A12 centre (101.3294, 134.5456) radius 1.005
  circle A13 centre (112.6906, 134.5456) radius 1.005
  circle A14 centre (121.3294, 134.5456) radius 1.005
  circle A15 centre (132.6906, 134.5456) radius 1.005
  circle A16 centre (141.3294, 134.5456) radius 1.005
  circle A17 centre (152.6906, 134.5456) radius 1.005
  circle A18 centre (161.3294, 134.5456) radius 1.005
  circle A19 centre (172.6906, 134.5456) radius 1.005
  circle A20 centre (94.4744, 96.3294) radius 1.005
  circle A21 centre (94.4744, 107.6906) radius 1.005
  circle A22 centre (94.4744, 116.3294) radius 1.005
  circle A23 centre (94.4744, 127.6906) radius 1.005
extrude "b back lines lines extrude Feature" add sketch "b back lines" along normal blind 3.175 separate body makes body 127
extrude "b back circles circles extrude Feature" add sketch "b back circles" along normal blind 3.175 separate body makes body 128 at (93.53, 116.6731, 2.1167) makes body 129 at (93.53, 96.6731, 2.1167) makes body 130 at (161.7427, 135.4617, 2.1167) makes body 131 at (141.7427, 135.4617, 2.1167) makes body 132 at (122.0992, 135.1916, 2.1167) makes body 133 at (102.0992, 135.1916, 2.1167) makes body 134 at (179.959, 128.6067, 2.1167) makes body 135 at (178.6013, 108.0344, 2.1167) makes body 136 at (171.7463, 89.8181, 2.1167) makes body 137 at (151.7463, 89.8181, 2.1167) makes body 138 at (131.7463, 89.8181, 2.1167) makes body 139 at (111.7463, 89.8181, 2.1167) makes body 140 at (120.385, 89.8181, 2.1167) makes body 141 at (140.385, 89.8181, 2.1167) makes body 142 at (160.385, 89.8181, 2.1167) makes body 143 at (178.6013, 96.6731, 2.1167) makes body 144 at (178.6013, 116.6731, 2.1167) makes body 145 at (100.385, 89.8181, 2.1167) makes body 146 at (113.4605, 135.1916, 2.1167) makes body 147 at (133.104, 135.4617, 2.1167) makes body 148 at (153.104, 135.4617, 2.1167) makes body 149 at (173.104, 135.4617, 2.1167) makes body 150 at (93.53, 108.0344, 2.1167) makes body 151 at (93.53, 128.0344, 2.1167)
combine "b back lines final combine feature" operation cut target body 127 tool bodies 128 129 130 131 132 133 134 135 136 137 138 139 140 141 142 143 144 145 146 147 148 149 150 151
hidden bodies 2 31 60 102 127
equation "d1163 = length"
equation "d1817 = depth"
equation "d289 = platformGrommetMountDiameter"
equation "d422 = length"
equation "d423 = depth"
equation "d843 = toolDiameter"
equation "d1634 = pcbMountHoles"
equation "d1797 = ( depth - 26 mm ) / 2"
equation "d1798 = ( length - 58 mm ) / 2"
equation "d492 = length"
equation "d493 = height"
equation "d502 = length"
equation "d503 = height"
equation "d230 = length"
equation "d231 = height"
equation "d1827 = depth"
equation "d1829 = ventDiameter"
equation "d910 = depth"
equation "d911 = height"
equation "d1819 = ventDiameter"
equation "b_ = 5 mm" comment "added by script"
equation "d467 = length"
equation "d468 = depth"
equation "d471 = ( depth - 26 mm ) / 2"
equation "d472 = ( length - 58 mm ) / 2"
equation "d479 = ventDiameter"
named bodies: "b  stockbody", "b top lines final body", "b top circles circle body", "b top circles circle body (1)", "b top circles circle body (2)", "b top circles circle body (3)", "b top circles circle body (4)", "b top circles circle body (5)", "b top circles circle body (6)", "b top circles circle body (7)", "b top circles circle body (8)", "b top circles circle body (9)", "b top circles circle body (10)", "b top circles circle body (11)", "b top circles circle body (12)", "b top circles circle body (13)", "b top circles circle body (14)", "b top circles circle body (15)", "b top circles circle body (16)", "b top circles circle body (17)", "b top circles circle body (18)", "b top circles circle body (19)", "b top circles circle body (20)", "b top circles circle body (21)", "b top circles circle body (22)", "b top circles circle body (23)", "b top circles circle body (24)", "b top circles circle body (25)", "b top circles circle body (26)", "b top circles circle body (27)", "b bottom lines final body", "b bottom circles circle body", "b bottom circles circle body (1)", "b bottom circles circle body (2)", "b bottom circles circle body (3)", "b bottom circles circle body (4)", "b bottom circles circle body (5)", "b bottom circles circle body (6)", "b bottom circles circle body (7)", "b bottom circles circle body (8)", "b bottom circles circle body (9)", "b bottom circles circle body (10)", "b bottom circles circle body (11)", "b bottom circles circle body (12)", "b bottom circles circle body (13)", "b bottom circles circle body (14)", "b bottom circles circle body (15)", "b bottom circles circle body (16)", "b bottom circles circle body (17)", "b bottom circles circle body (18)", "b bottom circles circle body (19)", "b bottom circles circle body (20)", "b bottom circles circle body (21)", "b bottom circles circle body (22)", "b bottom circles circle body (23)", "b bottom circles circle body (24)", "b bottom circles circle body (25)", "b bottom circles circle body (26)", "b bottom circles circle body (27)", "b left lines final body", "b left circles circle body", "b left circles circle body (1)", "b left circles circle body (2)", "b left circles circle body (3)", "b left circles circle body (4)", "b left circles circle body (5)", "b left circles circle body (6)", "b left circles circle body (7)", "b left circles circle body (8)", "b left circles circle body (9)", "b left circles circle body (10)", "b left circles circle body (11)", "b left circles circle body (12)", "b left circles circle body (13)", "b left circles circle body (14)", "b left circles circle body (15)", "b left circles circle body (16)", "b left circles circle body (17)", "b left circles circle body (18)", "b left circles circle body (19)", "b right lines final body", "b right circles circle body", "b right circles circle body (1)", "b right circles circle body (2)", "b right circles circle body (3)", "b right circles circle body (4)", "b right circles circle body (5)", "b right circles circle body (6)", "b right circles circle body (7)", "b right circles circle body (8)", "b right circles circle body (9)", "b right circles circle body (10)", "b right circles circle body (11)", "b right circles circle body (12)", "b right circles circle body (13)", "b right circles circle body (14)", "b right circles circle body (15)", "b right circles circle body (16)", "b right circles circle body (17)", "b right circles circle body (18)", "b right circles circle body (19)", "b front lines final body", "b front circles circle body", "b front circles circle body (1)", "b front circles circle body (2)", "b front circles circle body (3)", "b front circles circle body (4)", "b front circles circle body (5)", "b front circles circle body (6)", "b front circles circle body (7)", "b front circles circle body (8)", "b front circles circle body (9)", "b front circles circle body (10)", "b front circles circle body (11)", "b front circles circle body (12)", "b front circles circle body (13)", "b front circles circle body (14)", "b front circles circle body (15)", "b front circles circle body (16)", "b front circles circle body (17)", "b front circles circle body (18)", "b front circles circle body (19)", "b front circles circle body (20)", "b front circles circle body (21)", "b front circles circle body (22)", "b front circles circle body (23)", "b back lines final body", "b back circles circle body", "b back circles circle body (1)", "b back circles circle body (2)", "b back circles circle body (3)", "b back circles circle body (4)", "b back circles circle body (5)", "b back circles circle body (6)", "b back circles circle body (7)", "b back circles circle body (8)", "b back circles circle body (9)", "b back circles circle body (10)", "b back circles circle body (11)", "b back circles circle body (12)", "b back circles circle body (13)", "b back circles circle body (14)", "b back circles circle body (15)", "b back circles circle body (16)", "b back circles circle body (17)", "b back circles circle body (18)", "b back circles circle body (19)", "b back circles circle body (20)", "b back circles circle body (21)", "b back circles circle body (22)", "b back circles circle body (23)"
